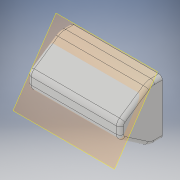
# Autodesk Inventor part: Part2
Saved by Autodesk Inventor 2018 (Build 220112000, 112)
## iProperties
Created: 2019-10-09
Part Number: Part2
Material: Generic
Document SubType Name: Modeling
Designer: Jacob
Density: 1 g/cm^3
Appearance: Default
Author: Jacob
Autodesk Inventor part; units mm, degrees
ref_plane "YZ Plane" through (0, 0, 0) normal (1, 0, 0) x (0, 1, 0)
ref_plane "XZ Plane" through (0, 0, 0) normal (0, 1, 0) x (-1, 0, 0)
ref_plane "XY Plane" through (0, 0, 0) normal (0, 0, 1) x (1, 0, 0)
sketch "Sketch1" plane through (0, 0, 0) normal (1, 0, 0) x (0, 1, 0)
  line L0 (-56, 44.45) -> (-56, -44.45) construction
  line L1 (-56, -44.45) -> (56, -44.45)
  line L2 (56, -44.45) -> (56, 44.45) construction
  line L3 (56, 44.45) -> (-56, -44.45) construction
  line L4 (-56, 44.45) -> (56, -44.45) construction
  line L5 (0, 0) -> (0, 44.45) construction
  line L6 (0, 44.45) -> (12.7, 44.45)
  line L7 (0, 44.45) -> (-12.7, 44.45)
  line L8 (56, -44.45) -> (12.7, 44.45)
  line L9 (-12.7, 44.45) -> (-56, -44.45)
  line L10 (56, -44.45) -> (56, -19.05)
  line L11 (56, -19.05) -> (12.7, 44.45)
  line L12 (-56, -44.45) -> (-56, -19.05)
  line L13 (-12.7, 44.45) -> (-56, -19.05)
  dimension "d0" = 112
  dimension "d1" = 88.9
  dimension "d2" = 12.7
  dimension "d3" = 12.7
  dimension "d13" = 25.4
  dimension "d14" = 25.4
  constraints: 28 end point, 2 horizontal, 2 midpoint, 2 point on line, 1 parallel, 1 vertical
  measures "d0" distance of L2.end L0.start
  measures "d1" distance of L1.end L2.end
  measures "d2" distance of L5.end L6.end
  measures "d3" distance of L7.end L5.end
  measures "d13" distance of L1.end L10.end
  measures "d14" distance of L0.end L12.end
extrude "Extrusion1" add sketch "Sketch1" along normal blind 195
shell "Shell1" thickness 6.35 outward yes removed faces 1 at (65, -18.6667, -44.45)
sketch "Sketch2" plane through (-6.35, -62.35, -44.45) normal (0, 0, -1) x (-1, 0, 0)
  line L0 (-207.7, 125.4132) -> (0, 125.4132)
  line L1 (0, 125.4132) -> (0, 0.7132)
  line L2 (0, 0.7132) -> (-207.7, 0.7132)
  line L3 (-207.7, 0.7132) -> (-207.7, 125.4132)
  line L4 (-201.35, 119.0632) -> (-6.35, 119.0632) projected
  line L5 (-6.35, 118.35) -> (-6.35, 6.35) projected
  line L6 (-6.35, 7.0632) -> (-201.35, 7.0632) projected
  line L7 (-201.35, 6.35) -> (-201.35, 118.35) projected
  line L8 (-238.3274, 162.0109) -> (68.8817, 162.0109)
  line L9 (68.8817, 162.0109) -> (68.8817, -36.1986)
  line L10 (68.8817, -36.1986) -> (-238.3274, -36.1986)
  line L11 (-238.3274, -36.1986) -> (-238.3274, 162.0109)
  point P0 (-6.35, 62.35)
  dimension "d7" = 6.35
  dimension "d8" = 6.35
  dimension "d9" = 6.35
  dimension "d10" = 6.35
  constraints: 16 end point, 4 parallel, 2 horizontal, 2 perpendicular
  measures "d7" distance between parallel lines of L0 L4
  measures "d8" distance between parallel lines of L1 L5
  measures "d9" distance between parallel lines of L2 L6
  measures "d10" distance between parallel lines of L7 L3
extrude "Extrusion2" cut sketch "Sketch2" against normal blind 195
fillet "Fillet4" radius 15 2 edges at (97.5, 16.0558, 50.8) (97.5, -16.0558, 50.8)
fillet "Fillet5" radius 8 14 edges at (-6.35, 62.35, -30.7705) (-6.35, 15.1373, 49.062) (-6.35, 0, 50.8) (-6.35, -15.1373, 49.062) (-6.35, -41.0793, 14.1027) (-6.35, 41.4359, 13.5798) (201.35, 62.35, -30.7705) (201.35, 15.1373, 49.062) (201.35, 0, 50.8) (201.35, -15.1373, 49.062) (201.35, -41.0793, 14.1027) (201.35, 41.4359, 13.5798) (-6.35, -61.6368, -30.2476) (201.35, -61.6368, -30.2476)
fillet "Fillet6" radius 30 8 edges at (97.5, -56, -19.05) (97.5, 56, -19.05) (199.0069, 60.0069, -17.8139) (-4.0069, 60.0069, -17.8139) (97.5, 62.35, -17.091) (199.0069, -59.2937, -16.768) (-4.0069, -59.2937, -16.768) (97.5, -61.6368, -16.0452)
ref_plane "Work Plane1" through (0, -12.7, 44.45) normal (0, 0.5633772, 0.8261998) x (1, 0, 0)
sketch "Sketch3" plane through (0, -12.7, 44.45) normal (0, 0.5633772, 0.8261998) x (1, 0, 0)
  point P0 (0, 35.5349)
body "Solid1"
